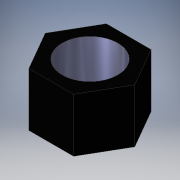
# Autodesk Inventor part: Three(mm)Nut
Saved by Autodesk Inventor 2016 (Build 200138000, 138)
## iProperties
Created: 2017-02-07
Part Number: Three(mm)Nut
Material: Generic
Document SubType Name: Modeling
Designer: Evan Phil George
Density: 1 g/cm^3
Appearance: Default
Author: Evan Phil George
Autodesk Inventor part; units mm, degrees
ref_plane "YZ Plane" through (0, 0, 0) normal (1, 0, 0) x (0, 1, 0)
ref_plane "XZ Plane" through (0, 0, 0) normal (0, 1, 0) x (-1, 0, 0)
ref_plane "XY Plane" through (0, 0, 0) normal (0, 0, 1) x (1, 0, 0)
sketch "Sketch1" plane through (0, 0, 0) normal (0, 1, 0) x (-1, 0, 0)
  circle A0 centre (0, 0) radius 1.55
  line L0 (-2.5, 0) -> (-1.25, 2.1651)
  line L1 (-1.25, 2.1651) -> (1.25, 2.1651)
  line L2 (1.25, 2.1651) -> (2.5, 0)
  line L3 (2.5, 0) -> (1.25, -2.1651)
  line L4 (1.25, -2.1651) -> (-1.25, -2.1651)
  line L5 (-1.25, -2.1651) -> (-2.5, 0)
  dimension "d0" = 3.1
  dimension "d1" = 2.5
  constraints: 12 end point, 2 coincident, 1 centre point, 13 other
  measures "d0" diameter of A0
  measures "d1" distance of L3.end L4.end
extrude "Extrusion1" add sketch "Sketch1" along normal blind 3
body "Solid1"
